Autodesk Inventor part; units mm, degrees
(part 2 of 2)
sketch "Sketch6" plane through (0, -65.8371, 0) normal (-1, 0, 0) x (0, 0, 1)
  circle A0 centre (2, 25.6685) radius 1.75 projected
  circle A1 centre (2, 35.6685) radius 1.75 projected
  line L0 (0, 43.4488) -> (4, 43.4488) projected
  line L1 (0, 43.4488) -> (0, 17.8883) projected
  line L2 (0, 17.8883) -> (4, 17.8883) projected
  line L3 (4, 43.4488) -> (4, 17.8883) projected
  point P0 (0, 65.8371)
hole "Hole4" at (0, -40.1685, 2) at (0, -30.1685, 2) direction (1, 0, 0) diameter 2.9 end through all countersink diameter 6 countersink angle 90 clearance for "Countersunk Flat Head Screw ISO 2009/7046" size "M2.5" standard "ISO"
body "Solid1"
